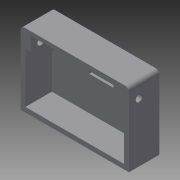
# Autodesk Inventor part: Case_Cutout
Saved by Autodesk Inventor 2014 (Build 180170000, 170)
## iProperties
Created: 2014-05-02
Part Number: Case_Cutout
Material: Generic
Document SubType Name: Modeling
Designer: Alex
Density: 1 g/cm^3
Appearance: Default
Author: Alex
Autodesk Inventor part; units mm, degrees
ref_plane "YZ Plane" through (0, 0, 0) normal (1, 0, 0) x (0, 1, 0)
ref_plane "XZ Plane" through (0, 0, 0) normal (0, 1, 0) x (-1, 0, 0)
ref_plane "XY Plane" through (0, 0, 0) normal (0, 0, 1) x (1, 0, 0)
sketch "Sketch1" plane through (0, 0, 0) normal (0, 0, 1) x (1, 0, 0)
  line L0 (0, 0) -> (68.58, 0)
  line L1 (68.58, 0) -> (68.58, 46.228)
  line L2 (68.58, 46.228) -> (0, 46.228)
  line L3 (0, 46.228) -> (0, 0)
  dimension "d0" = 68.58
  dimension "d1" = 46.228
  constraints: 8 end point, 2 parallel, 1 horizontal, 1 perpendicular
  measures "d0" distance of L1.end L2.end
  measures "d1" distance of L2.end L0.start
extrude "Extrusion1" add sketch "Sketch1" along normal blind 2.54
sketch "Sketch2" plane through (0, 0, 2.54) normal (0, 0, 1) x (1, 0, 0)
  line L0 (0, 46.228) -> (0, 0) projected
  line L1 (0, 46.228) -> (68.58, 46.228)
  line L2 (68.58, 46.228) -> (68.58, 0)
  line L3 (68.58, 0) -> (0, 0)
  line L4 (0, 0) -> (0, 46.228)
  line L5 (6.35, 43.688) -> (59.69, 43.688)
  line L6 (59.69, 43.688) -> (59.69, 28.448)
  line L7 (59.69, 28.448) -> (6.35, 28.448)
  line L8 (6.35, 28.448) -> (6.35, 43.688)
  line L9 (3.048, 28.448) -> (65.532, 28.448)
  line L10 (65.532, 28.448) -> (65.532, 3.048)
  line L11 (65.532, 3.048) -> (3.048, 3.048)
  line L12 (3.048, 3.048) -> (3.048, 28.448)
  dimension "d4" = 62.484
  dimension "d5" = 53.34
  dimension "d6" = 15.24
  dimension "d7" = 25.4
  dimension "d8" = 3.048
  dimension "d9" = 3.048
  dimension "d10" = 0
  dimension "d13" = 6.35
  constraints: 24 end point, 6 parallel, 3 horizontal, 3 perpendicular
  measures "d4" distance of L10.end L11.end
  measures "d5" distance of L5.start L5.end
  measures "d6" distance of L7.end L5.start
  measures "d7" distance of L11.end L9.start
  measures "d8" distance between parallel lines of L3 L11
  measures "d9" distance between parallel lines of L0 L12
  measures "d10" distance between parallel lines of L9 L7
  measures "d13" distance between parallel lines of L0 L8
extrude "Extrusion2" add sketch "Sketch2" along normal blind 16.764
chamfer "Chamfer1" distance 6.35 distance2 12.7 1 edges at (62.611, 28.448, 19.304) measured on face at (23.876, 1.016, 19.304)
chamfer "Chamfer2" distance 6.35 distance2 12.7 1 edges at (4.699, 28.448, 19.304) measured on face at (23.876, 1.016, 19.304)
sketch "Sketch3" plane through (0, 0, 2.54) normal (0, 0, 1) x (1, 0, 0)
  circle A0 centre (34.29, 36.068) radius 3.4925
  line L0 (0, 0) -> (68.58, 0) projected
  line L1 (0, 46.228) -> (0, 0) projected
  line L2 (68.58, 46.228) -> (0, 46.228) projected
  line L3 (68.58, 0) -> (68.58, 46.228) projected
  dimension "d22" = 10.16
  dimension "d23" = 34.29
  dimension "d24" = 6.985
  constraints: 1 centre point
  measures "d22" distance from line of L2 A0.centre
  measures "d23" distance from line of L1 A0.centre
  measures "d24" diameter of A0
extrude "Extrusion3" cut sketch "Sketch3" against normal up to surface (2.54 mm away) contours A0
sketch "Sketch4" plane through (0, 0, 2.54) normal (0, 0, 1) x (1, 0, 0)
  line L0 (59.69, 28.448) -> (59.69, 43.688) projected
  line L1 (59.69, 43.688) -> (6.35, 43.688) projected
  circle A0 centre (44.704, 36.068) radius 1.4732
  point P0 (0, 0)
  dimension "d27" = 2.9464
  dimension "d28" = 7.62
  dimension "d29" = 14.986
  constraints: 1 centre point
  measures "d27" diameter of A0
  measures "d28" distance from line of L1 A0.centre
  measures "d29" distance from line of L0 A0.centre
extrude "Extrusion4" add sketch "Sketch4" along normal blind 7.62
fillet "Fillet1" radius 1.4732 1 edges at (43.2308, 36.068, 10.16)
fillet "Fillet2" radius 2.54 2 edges at (0, 46.228, 9.652) (68.58, 46.228, 9.652)
sketch "Sketch5" plane through (0, 0, 2.54) normal (0, 0, 1) x (1, 0, 0)
  circle A0 centre (34.29, 36.068) radius 3.4925 projected
  line L0 (26.67, 43.688) -> (41.91, 43.688)
  line L1 (41.91, 43.688) -> (41.91, 24.638)
  line L2 (41.91, 24.638) -> (26.67, 24.638)
  line L3 (26.67, 24.638) -> (26.67, 43.688)
  point P0 (0, 0)
  dimension "d34" = 19.05
  dimension "d35" = 15.24
  dimension "d36" = 7.62
  dimension "d37" = 7.62
  constraints: 8 end point, 2 parallel, 1 horizontal, 1 perpendicular
  measures "d34" distance of L2.end L0.start
  measures "d35" distance of L1.end L2.end
  measures "d36" distance from line of L0 A0.centre
  measures "d37" distance from line of A0.centre L1
extrude "Extrusion5" cut sketch "Sketch5" against normal blind 1.524
hole "Hole1" at (68.58, 37.338, 12.954) direction (-1, 0, 0) diameter 4.1656 end through all
equation "\"d9\" = d8"
body "Solid1"
